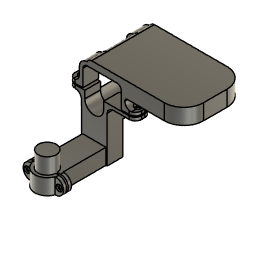
ENSAMBLE_MONITOR v5 (Autodesk Fusion 360 design; units mm, degrees)
Autodesk Fusion 360 part; units mm, degrees
sketch "Boceto1" plane through (0, 0, 0) normal (0, 1, 0) x (-1, 0, 0)
  line L0 (5, 46.2017) -> (43, 46.2017)
  line L1 (48, 41.2017) -> (48, 20.2017)
  line L2 (48, 20.2017) -> (0, 20.2017)
  line L3 (0, 20.2017) -> (0, 41.2017)
  arc A0 (48, 41.2017) -> (43, 46.2017) centre (43, 41.2017) ccw
  arc A1 (5, 46.2017) -> (0, 41.2017) centre (5, 41.2017) ccw
  circle A2 centre (34, 8.7017) radius 11.5
  point P0 (0, 46.2017)
  point P1 (48, 46.2017)
  dimension "d1" = 48
  dimension "d2" = 26
  dimension "d3" = 5
  dimension "d4" = 5
  dimension "d7" = 23
  dimension "d41" = 14
  constraint horizontal L0
  constraint vertical L1
  constraint horizontal L2
  constraint vertical L3
  constraint coincident P1 L0
  constraint coincident P1 L1
  constraint tangent L0 A0
  constraint tangent L1 A0
  constraint coincident P0 L0
  constraint coincident P0 L3
  constraint tangent L0 A1
  constraint tangent L3 A1
  constraint tangent L2 A2
  measures "d1" distance of P0 P1
  measures "d2" distance of P0 L2.end
  measures "d3" radius of A0
  measures "d4" radius of A1
  measures "d7" diameter of A2
  measures "d41" horizontal distance of L1.end A2.centre
extrude "Extruir1" add sketch "Boceto1" along normal blind 100 makes body 1
sketch "Boceto2" plane through (0, 0, 0) normal (0, -1, 0) x (1, 0, 0)
  arc A0 (-43, 46.2017) -> (-48, 41.2017) centre (-43, 41.2017) ccw
  line L0 (-48, 41.2017) -> (-48, 20.2017)
  line L1 (-48, 20.2017) -> (-34, 20.2017)
  line L2 (-34, 20.2017) -> (0, 20.2017)
  line L3 (0, 20.2017) -> (0, 41.2017)
  arc A1 (0, 41.2017) -> (-5, 46.2017) centre (-5, 41.2017) ccw
  line L4 (-5, 46.2017) -> (-43, 46.2017)
  circle A2 centre (-34, 8.7017) radius 11.5
  line L5 (-48.5, 41.2017) -> (-48.5, 19.7017)
  line L6 (-48.5, 19.7017) -> (-31.5, 19.7017)
  line L7 (-31.5, 19.7017) -> (0.5, 19.7017)
  line L8 (0.5, 19.7017) -> (0.5, 41.2017)
  arc A3 (0.5, 41.2017) -> (-5, 46.7017) centre (-5, 41.2017) ccw
  line L9 (-5, 46.7017) -> (-43, 46.7017)
  arc A4 (-43, 46.7017) -> (-48.5, 41.2017) centre (-43, 41.2017) ccw
  circle A5 centre (-34, 8.7017) radius 12
  line L10 (-53, 41.2017) -> (-53, 15.2017)
  line L11 (-53, 15.2017) -> (-31.5, 15.2017)
  line L12 (-31.5, 15.2017) -> (5, 15.2017)
  line L13 (5, 15.2017) -> (5, 41.2017)
  arc A6 (5, 41.2017) -> (-5, 51.2017) centre (-5, 41.2017) ccw
  line L14 (-5, 51.2017) -> (-43, 51.2017)
  arc A7 (-43, 51.2017) -> (-53, 41.2017) centre (-43, 41.2017) ccw
  line L15 (-48.5, 19.7017) -> (-66.5, 19.7017)
  line L16 (-66.5, 19.7017) -> (-66.5, 23.7017)
  line L17 (-66.5, 23.7017) -> (-48.5, 23.7017)
  line L18 (-48.5, 23.7017) -> (-48.5, 19.7017)
  line L19 (0.5, 19.7017) -> (18.5, 19.7017)
  line L20 (18.5, 19.7017) -> (18.5, 23.7017)
  line L21 (18.5, 23.7017) -> (0.5, 23.7017)
  line L22 (0.5, 23.7017) -> (0.5, 19.7017)
  circle A8 centre (-34, 8.7017) radius 16.5
  line L23 (18.5, 19.7017) -> (18.5, -0.2983) construction
  line L24 (-66.5, 19.7017) -> (-66.5, -0.2983) construction
  line L25 (-66.5, 18.2017) -> (-44.6654, 18.2017)
  line L26 (-44.6654, 18.2017) -> (-44.6654, 14.2017)
  line L27 (-44.6654, 14.2017) -> (-66.5, 14.2017)
  line L28 (-66.5, 14.2017) -> (-66.5, 18.2017)
  line L29 (-23.3346, 14.2017) -> (18.5, 14.2017)
  line L30 (18.5, 14.2017) -> (18.5, 18.2017)
  line L31 (18.5, 18.2017) -> (-23.3346, 18.2017)
  line L32 (-23.3346, 18.2017) -> (-23.3346, 14.2017)
  line L33 (-46, 8.7017) -> (-46, 18.2017)
  line L34 (-22, 8.7017) -> (-22, 18.2017)
  dimension "d9" = 0.5
  dimension "d10" = 0.5
  dimension "d11" = 5
  dimension "d12" = 18
  dimension "d13" = 4
  dimension "d14" = 18
  dimension "d15" = 4
  dimension "d16" = 5
  dimension "d17" = 20
  dimension "d18" = 20
  dimension "d19" = 1.5
  dimension "d20" = 4
  dimension "d21" = 1.5
  dimension "d22" = 4
  constraint horizontal L15
  constraint vertical L16
  constraint horizontal L17
  constraint vertical L18
  constraint horizontal L19
  constraint vertical L20
  constraint horizontal L21
  constraint vertical L22
  constraint perpendicular L19 L23
  constraint perpendicular L15 L24
  constraint horizontal L25
  constraint vertical L26
  constraint horizontal L27
  constraint vertical L28
  constraint coincident A5 L26.end
  constraint coincident L24 L25.start
  constraint horizontal L29
  constraint vertical L30
  constraint horizontal L31
  constraint vertical L32
  constraint coincident L23 L30.end
  constraint coincident A5 L29.start
  constraint coincident A5 L33.start
  constraint coincident L25 L33.end
  constraint tangent A5 L33
  constraint vertical L33
  constraint coincident A5 L34.start
  constraint coincident L31 L34.end
  constraint perpendicular L31 L34
  constraint tangent A5 L34
  measures "d12" distance of L16.end L17.end
  measures "d13" distance of L15.end L16.end
  measures "d14" distance of L20.end L21.end
  measures "d15" distance of L19.end L20.end
  measures "d17" distance of L15.end L24.end
  measures "d18" distance of L19.end L23.end
  measures "d19" distance of L15 L25
  measures "d20" distance of L25.end L26.end
  measures "d21" distance of L19 L31
  measures "d22" distance of L29.start L31.end
extrude "Extruir2" add sketch "Boceto2" against normal blind 20 separate body contours L5 L10 L15 L17 L18 | L8 L13 L19 L21 L22 | L5 L8 A3 L9 A4 L10 L13 A6 L14 A7 L17 L21 | L10 L15 L16 L17 | L13 L19 L20 L21 makes body 2
extrude "Extruir3" add sketch "Boceto2" against normal blind 20 separate body contours L11 A8 L25 L33 | L10 L11 A8 L25 | L12 L13 A8 L31 | L12 A8 L31 L34 | L10 L11 A8 L25 L27 L28 | L11 A8 L27 L33 | L12 A8 L29 L34 | L12 L13 A8 L29 L30 L31 | A5 A8 L27 L29 L33 L34 makes body 3
fillet "Empalme1" radius 8 8 edges at (-66.5, 0, 21.7017) (-66.5, 20, 21.7017) (18.5, 0, 21.7017) (18.5, 20, 21.7017) (-66.5, 0, 16.2017) (-66.5, 20, 16.2017) (18.5, 0, 16.2017) (18.5, 20, 16.2017) on bodies 2 3
sketch "Boceto3" plane through (0, 0, 23.7017) normal (0, 0, 1) x (-1, 0, 0)
  arc A0 (58.5, -20) -> (66.5, -12) centre (58.5, -12) ccw
  line L0 (66.5, -12) -> (66.5, -8)
  arc A1 (66.5, -8) -> (58.5, 0) centre (58.5, -8) ccw
  line L1 (58.5, 0) -> (53, 0)
  line L2 (53, 0) -> (53, -20)
  line L3 (53, -20) -> (58.5, -20)
  arc A2 (-18.5, -12) -> (-10.5, -20) centre (-10.5, -12) ccw
  line L4 (-10.5, -20) -> (-5, -20)
  line L5 (-5, -20) -> (-5, 0)
  line L6 (-5, 0) -> (-10.5, 0)
  arc A3 (-10.5, 0) -> (-18.5, -8) centre (-10.5, -8) ccw
  line L7 (-18.5, -8) -> (-18.5, -12)
  line L8 (53, -10) -> (66.5, -10) construction
  line L9 (-5, -10) -> (-18.5, -10) construction
  circle A4 centre (59.75, -10) radius 2.125
  circle A5 centre (59.75, -10) radius 4
  circle A6 centre (-11.75, -10) radius 2.125
  circle A7 centre (-11.75, -10) radius 4
  dimension "d29" = 4.25
  dimension "d30" = 8
  dimension "d31" = 4.25
  dimension "d32" = 8
  constraint midpoint L2 L8.start
  constraint midpoint L0 L8.end
  constraint midpoint L5 L9.start
  constraint midpoint L7 L9.end
  constraint midpoint L8 A4.centre
  constraint concentric A4 A5
  constraint midpoint L9 A6.centre
  constraint concentric A6 A7
  measures "d29" diameter of A4
  measures "d30" diameter of A5
  measures "d31" diameter of A6
  measures "d32" diameter of A7
extrude "Extruir4" cut sketch "Boceto3" against normal blind 9.5 contours A4 | A6 bodies 2 3
extrude "Extruir5" cut sketch "Boceto3" against normal blind 2 contours A5 | A7 bodies 2
sketch "Boceto4" plane through (0, 0, 14.2017) normal (0, 0, -1) x (1, 0, 0)
  circle A0 centre (-59.75, -10) radius 2.125
  arc A1 (-66.5, -12) -> (-58.5, -20) centre (-58.5, -12) ccw
  line L0 (-58.5, -20) -> (-49.5563, -20)
  line L1 (-49.5563, -20) -> (-49.5563, 0)
  line L2 (-49.5563, 0) -> (-58.5, 0)
  arc A2 (-58.5, 0) -> (-66.5, -8) centre (-58.5, -8) ccw
  line L3 (-66.5, -8) -> (-66.5, -12)
  circle A3 centre (11.75, -10) radius 4
  circle A4 centre (-59.75, -10) radius 4
extrude "Extruir6" cut sketch "Boceto4" against normal blind 2 contours A3 | A4 bodies 3
fillet "Empalme2" radius 8 4 edges at (5, 10, 23.7017) (-53, 10, 23.7017) (-18.4437, 10, 14.2017) (-49.5563, 10, 14.2017) on bodies 2 3
copy_body "CopiarPegarCuerpos1" bodies 2 3 makes body 4 makes body 5
move_body "Desplazar1" bodies 4 5 to x (1, 0, 0) y (0, 1, 0) z (0, 0, 1) at (0, 60, 0)
sketch "Boceto5" plane through (0, 0, 0) normal (0, -1, 0) x (1, 0, 0)
  line L0 (10.5, 19.7017) -> (10.5, 24.1024)
  arc A0 (5, 31.7017) -> (10.5, 24.1024) centre (13, 31.7017) ccw
  line L1 (5, 31.7017) -> (5, 41.2017)
  arc A1 (5, 41.2017) -> (-5, 51.2017) centre (-5, 41.2017) ccw
  line L2 (-5, 51.2017) -> (-43, 51.2017)
  arc A2 (-43, 51.2017) -> (-53, 41.2017) centre (-43, 41.2017) ccw
  line L3 (-53, 41.2017) -> (-53, 31.7017)
  arc A3 (-58.5, 24.1024) -> (-53, 31.7017) centre (-61, 31.7017) ccw
  line L4 (-58.5, 24.1024) -> (-58.5, 19.7017)
  line L5 (-58.5, 19.7017) -> (-48.5, 19.7017)
  line L6 (-48.5, 19.7017) -> (-48.5, 41.2017)
  arc A4 (-43, 46.7017) -> (-48.5, 41.2017) centre (-43, 41.2017) ccw
  line L7 (-43, 46.7017) -> (-5, 46.7017)
  arc A5 (0.5, 41.2017) -> (-5, 46.7017) centre (-5, 41.2017) ccw
  line L8 (0.5, 41.2017) -> (0.5, 19.7017)
  line L9 (0.5, 19.7017) -> (10.5, 19.7017)
  line L10 (-43, 51.2017) -> (80.5, 51.2017)
  line L11 (80.5, 51.2017) -> (80.5, 55.2017)
  line L12 (80.5, 55.2017) -> (-43, 55.2017)
  line L13 (-43, 55.2017) -> (-43, 51.2017)
  line L14 (80.5, 51.2017) -> (0.5, 51.2017)
  line L15 (0.5, 51.2017) -> (0.5, 35.2017)
  line L16 (0.5, 35.2017) -> (80.5, 35.2017)
  line L17 (80.5, 35.2017) -> (80.5, 51.2017)
  arc A6 (5, 41.2017) -> (-5, 51.2017) centre (-5, 41.2017) ccw
  dimension "d42" = 4
  dimension "d43" = 20
  dimension "d53" = 80
  constraint horizontal L10
  constraint vertical L11
  constraint horizontal L12
  constraint vertical L13
  constraint coincident L2.end A2.start
  constraint horizontal L14
  constraint vertical L15
  constraint horizontal L16
  constraint vertical L17
  constraint coincident L8 L15.end
  measures "d42" distance of L2.end L12.end
  measures "d43" distance of L12 L16
  measures "d53" distance of L15 L17
extrude "Extruir7" add sketch "Boceto5" against normal blind 80 contours L1 A1 L10 L14 L15 L16 L17 A6 | A1 L10 L15 A6 | L2 L10 L11 L12 L13 L14 bodies 2 4
fillet "Empalme3" radius 3 2 edges at (5, 10, 35.2017) (5, 70, 35.2017) on bodies 2
fillet "Empalme4" radius 6 1 edges at (-43, 40, 55.2017) on bodies 2
fillet "Empalme5" radius 25 2 edges at (80.5, 0, 45.2017) (80.5, 80, 45.2017) on bodies 2
ref_plane "PlanoDeObra1" through (-45.5, 37.9312, 8.7017) normal (-1, 0, 0) x (0, 0, -1)
sketch "Boceto6" plane through (-45.5, 0, 0) normal (-1, 0, 0) x (0, -1, 0)
  line L0 (0, 20.2017) -> (0, -2.7983)
  line L1 (0, 8.7017) -> (60, 8.7017) construction
  line L2 (60, 8.7017) -> (60, -51.2983) construction
  line L3 (60, -51.2983, 0) -> (60, -51.2983, -11.5) construction
  circle A0 through (48.5, -51.2983, -11.5) (65.75, -51.2983, -1.5407) (65.75, -51.2983, -21.4593)
  dimension "d55" = 60
  dimension "d56" = 60
  dimension "d57" = 11.5
  dimension "d58" = 23
  constraint midpoint L0 L1.start
  constraint perpendicular L0 L1
  constraint perpendicular L1 L2
  measures "d55" distance of L1.start L1.end
  measures "d56" distance of L1.end L2.end
extrude "Extruir8" add sketch "Boceto6" along normal blind 40 separate body contours A0 in plane through (-45.5, 0, -51.2983) normal (0, 0, 1) makes body 6
sketch "Boceto7" plane through (0, 0, -51.2983) normal (0, 0, -1) x (1, 0, 0)
  circle A0 centre (-34, 60) radius 11.5
  circle A1 centre (-34, 60) radius 11.8
  circle A2 centre (-34, 60) radius 15.8
  line L0 (-34, 60) -> (-18.2, 60)
  line L1 (-34, 60) -> (-49.8, 60)
  line L2 (-49.8, 61) -> (-18.2, 61)
  line L3 (-18.2, 61) -> (-18.2, 59)
  line L4 (-18.2, 59) -> (-49.8, 59)
  line L5 (-49.8, 59) -> (-49.8, 61)
  line L6 (-45.8, 61) -> (-59.8, 61)
  line L7 (-59.8, 61) -> (-59.8, 65)
  line L8 (-59.8, 65) -> (-45.8, 65)
  line L9 (-45.8, 65) -> (-45.8, 61)
  line L10 (-22.2424, 61) -> (-8.2424, 61)
  line L11 (-8.2424, 61) -> (-8.2424, 65)
  line L12 (-8.2424, 65) -> (-22.2424, 65)
  line L13 (-22.2424, 65) -> (-22.2424, 61)
  dimension "d61" = 0.3
  dimension "d62" = 4
  dimension "d64" = 1
  dimension "d65" = 1
  dimension "d67" = 14
  dimension "d68" = 4
  dimension "d69" = 4
  dimension "d70" = 14
  constraint concentric A0 A1
  constraint concentric A0 A2
  constraint coincident A0.centre A1.centre
  constraint coincident A2 L0.end
  constraint horizontal L0
  constraint parallel L0 L1
  constraint horizontal L2
  constraint perpendicular L2 L3
  constraint perpendicular L3 L4
  constraint perpendicular L2 L5
  constraint tangent A2 L5
  constraint tangent A2 L3
  constraint horizontal L6
  constraint vertical L7
  constraint horizontal L8
  constraint vertical L9
  constraint coincident L2 L6.start
  constraint horizontal L10
  constraint vertical L11
  constraint horizontal L12
  constraint vertical L13
  constraint coincident A1 L10.start
  constraint coincident L2 L10.start
  constraint tangent A1 L9
  measures "d61" distance of A0 A1
  measures "d62" distance of A1 A2
  measures "d64" distance of L1 L2
  measures "d65" distance of L1 L4
  measures "d67" distance of L7 L9
  measures "d68" distance of L6.end L7.end
  measures "d69" distance of L10.end L11.end
  measures "d70" distance of L11.end L12.end
extrude "Extruir9" add sketch "Boceto7" against normal blind 20 separate body contours A2 L2 L10 L12 L13 | A1 A2 L2 L8 L9 L12 L13 | A2 L2 L10 L11 L12 | A2 L2 L6 L8 L9 | A2 L2 L6 L7 L8 makes body 7
sketch "Boceto8" plane through (0, -65, 0) normal (0, -1, 0) x (1, 0, 0)
  line L0 (-59.8, -51.2983) -> (-48.988, -51.2983)
  line L1 (-48.988, -51.2983) -> (-48.988, -31.2983)
  line L2 (-48.988, -31.2983) -> (-59.8, -31.2983)
  line L3 (-59.8, -31.2983) -> (-59.8, -51.2983)
  line L4 (-54.394, -31.2983) -> (-54.394, -51.2983) construction
  line L5 (-19.012, -31.2983) -> (-8.2424, -31.2983) construction
  line L6 (-8.2424, -51.2983) -> (-19.012, -51.2983) construction
  line L7 (-13.6272, -31.2983) -> (-13.6272, -51.2983) construction
  circle A0 centre (-54.394, -41.2983) radius 2.125
  line L8 (-19.012, -51.2983) -> (-8.2424, -51.2983)
  line L9 (-8.2424, -51.2983) -> (-8.2424, -31.2983)
  line L10 (-8.2424, -31.2983) -> (-19.012, -31.2983)
  line L11 (-19.012, -31.2983) -> (-19.012, -51.2983)
  circle A1 centre (-13.6272, -41.2983) radius 2.125
  circle A2 centre (-13.6272, -41.2983) radius 4
  circle A3 centre (-54.394, -41.2983) radius 4
  dimension "d73" = 4.25
  dimension "d75" = 4.25
  dimension "d76" = 8
  dimension "d77" = 8
  constraint midpoint L2 L4.start
  constraint midpoint L0 L4.end
  constraint midpoint L5 L7.start
  constraint midpoint L6 L7.end
  constraint midpoint L4 A0.centre
  constraint midpoint L7 A1.centre
  constraint concentric A1 A2
  constraint concentric A0 A3
  measures "d73" diameter of A0
  measures "d75" diameter of A1
  measures "d76" diameter of A2
  measures "d77" diameter of A3
fillet "Empalme6" radius 10 4 edges at (-59.8, -63, -31.2983) (-59.8, -63, -51.2983) (-8.2424, -63, -31.2983) (-8.2424, -63, -51.2983) on bodies 7
extrude "Extruir10" cut sketch "Boceto8" against normal blind 2 contours A0 | A1 | A2 | A3 bodies 7
extrude "Extruir11" cut sketch "Boceto8" against normal blind 4 contours A0 | A1 bodies 7
copy_body "CopiarPegarCuerpos2" bodies 7 makes body 8
move_body "Desplazar2" bodies 8 to x (-1, 0, 0) y (0, -1, 0) z (0, 0, 1) at (-119.6, -151.6, 0)
move_body "Desplazar3" bodies 8 to x (1, 0, 0) y (0, 1, 0) z (0, 0, 1) at (51.6, 19.8, -20)
move_body "Desplazar4" bodies 8 to x (1, 0, 0) y (0, 1, 0) z (0, 0, 1) at (0, 15, 20)
move_body "Desplazar5" bodies 8 to x (1, 0, 0) y (0, 1, 0) z (0, 0, 1) at (0, -15, 0)
move_body "Desplazar6" bodies 8 to x (1, 0, 0) y (0, 1, 0) z (0, 0, 1) at (0, 12, 0)
ref_plane "PlanoDeObra2" through (-34, 10.6908, -7.7983) normal (0, 0, -1) x (1, 0, 0)
sketch "Boceto10" plane through (0, 80, 0) normal (0, 1, 0) x (-1, 0, 0)
  line L0 (-10.5, 18.2017) -> (-10.5, 14.2017)
  line L1 (-10.5, 14.2017) -> (9.6279, 14.2017)
  arc A0 (17.5861, 7.0181) -> (9.6279, 14.2017) centre (9.6279, 6.2017) ccw
  arc A1 (17.5861, 7.0181) -> (50.4139, 7.0181) centre (34, 8.7017) ccw
  arc A2 (58.3721, 14.2017) -> (50.4139, 7.0181) centre (58.3721, 6.2017) ccw
  line L2 (58.3721, 14.2017) -> (58.5, 14.2017)
  line L3 (58.5, 14.2017) -> (58.5, 18.2017)
  line L4 (58.5, 18.2017) -> (46, 18.2017)
  line L5 (46, 18.2017) -> (46, 8.7017)
  arc A3 (22, 8.7017) -> (46, 8.7017) centre (34, 8.7017) ccw
  line L6 (22, 8.7017) -> (22, 18.2017)
  line L7 (22, 18.2017) -> (-10.5, 18.2017)
  line L8 (17.5861, 7.0181) -> (17.5861, -9.2983)
  line L9 (17.5861, -9.2983) -> (50.1072, -9.2983)
  line L10 (50.1072, -9.2983) -> (50.4139, 7.0181)
  dimension "d90" = 18
  constraint coincident A0.start A1.start
  constraint vertical L8
  constraint perpendicular L8 L9
  constraint coincident A1.end A2.end
  measures "d90" distance of A1.centre L9
extrude "Extruir13" add sketch "Boceto10" against normal blind 80 contours A1 L8 L9 L10 bodies 3 5
sketch "Boceto12" plane through (0, 0, -51.2983) normal (0, 0, -1) x (1, 0, 0)
  line L0 (-49.7576, 58.8) -> (-49.7576, 54.8)
  line L1 (-49.7576, 54.8) -> (-48.988, 54.8)
  arc A0 (-48.988, 54.8) -> (-19.012, 54.8) centre (-34, 59.8) ccw
  line L2 (-19.012, 54.8) -> (-18.2, 54.8)
  line L3 (-18.2, 54.8) -> (-18.2, 58.8)
  line L4 (-18.2, 58.8) -> (-22.2, 58.8)
  line L5 (-22.2, 58.8) -> (-22.2424, 58.8)
  arc A1 (-45.7576, 58.8) -> (-22.2424, 58.8) centre (-34, 59.8) ccw
  line L6 (-45.7576, 58.8) -> (-49.7576, 58.8)
  line L7 (-19.012, 54.8) -> (-19.012, 42.8)
  line L8 (-19.012, 42.8) -> (-48.988, 42.8)
  line L9 (-48.988, 42.8) -> (-48.988, 54.8)
  line L10 (-49.7576, 54.8) -> (-59.7576, 54.8)
  dimension "d93" = 12
  constraint coincident A0.end L2.start
  constraint perpendicular L2 L7
  constraint perpendicular L0 L8
  constraint coincident L1.end A0.start
  constraint vertical L9
  measures "d93" distance of L8 L10
extrude "Extruir14" add sketch "Boceto12" against normal blind 20 contours A0 L7 L8 L9 bodies 8
move_body "Desplazar7" bodies 8 7 to x (1, 0, 0) y (0, 1, 0) z (0, 0, 1) at (0, 0, 10)
move_body "Desplazar8" bodies 7 8 to x (1, 0, 0) y (0, 1, 0) z (0, 0, 1) at (0, 0, -10)
extrude "Extruir15" add 1 faces at (-29.004, -42.8, -44.6316) along direction (0, 1, 0) blind 42.8 on bodies 8 bodies 8
sketch "Boceto13" plane through (0, 0, -9.2983) normal (0, 0, -1) x (1, 0, 0)
  line L0 (-50.1072, -80) -> (-17.5861, -80)
  line L1 (-17.5861, -80) -> (-17.5861, 0)
  line L2 (-17.5861, 0) -> (-50.1072, 0)
  line L3 (-50.1072, 0) -> (-50.1072, -80)
  line L4 (-50.1072, 0) -> (-17.5861, 0)
  line L5 (-17.5861, 0) -> (-17.5861, -20)
  line L6 (-17.5861, -20) -> (-50.1072, -20)
  line L7 (-50.1072, -20) -> (-50.1072, 0)
  dimension "d98" = 20
  constraint horizontal L4
  constraint vertical L5
  constraint horizontal L6
  constraint vertical L7
  constraint coincident L1 L5.end
  constraint coincident L2.end L3.start
  measures "d98" distance of L2.end L6.end
extrude "Extruir16" add sketch "Boceto13" along normal blind 42 contours L1 L2 L3 L4 L5 L6 L7 bodies 3 8
fillet "Empalme7" [suppressed]
fillet "Empalme8" [suppressed]
hidden bodies 1
equation "d57 = ( 23 / 2 ) * 1 mm"
named bodies: "SUP_C", "INF_C", "SUP_C (1)", "INF_C (1)"
